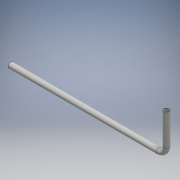
# Autodesk Inventor part: Tube
Saved by Autodesk Inventor 2016 (Build 200138000, 138)
## iProperties
Created: 2016-12-04
Part Number: Tube
Material: Generic
Document SubType Name: Modeling
Designer: Muhammad
Density: 1 g/cm^3
Appearance: Default
Author: Muhammad
Autodesk Inventor part; units mm, degrees
ref_plane "YZ Plane" through (0, 0, 0) normal (1, 0, 0) x (0, 1, 0)
ref_plane "XZ Plane" through (0, 0, 0) normal (0, 1, 0) x (-1, 0, 0)
ref_plane "XY Plane" through (0, 0, 0) normal (0, 0, 1) x (1, 0, 0)
sketch "Sketch1" plane through (0, 0, 0) normal (0, 1, 0) x (-1, 0, 0)
  line L0 (0, 0) -> (-166.5, 0)
  line L1 (-166.5, 0) -> (-166.5, 8.5) construction
  arc A0 (-175, 8.5) -> (-166.5, 0) centre (-166.5, 8.5) ccw
  line L2 (-175, 8.5) -> (-175, 43.681)
  dimension "d1" = 8.5
  dimension "d2" = 35.181
  constraints: 6 end point, 2 point on circle, 2 vertical, 1 centre point, 1 coincident, 1 horizontal
  measures "d1" distance of L0.end L1.end
  measures "d2" distance of L2.start L2.end
sketch "Sketch2" plane through (0, 0, 0) normal (1, 0, 0) x (0, 1, 0)
  circle A0 centre (0, 0) radius 3
  circle A1 centre (0, 0) radius 2.5
  dimension "d3" = 6
  dimension "d4" = 5
  constraints: 2 centre point, 2 coincident
  measures "d3" diameter of A0
  measures "d4" diameter of A1
sweep "Sweep1" add profiles "Sketch2" path "Sketch1"
body "Solid1"
